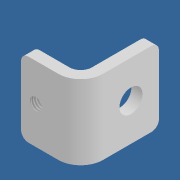
# Autodesk Inventor part: Belt_Tenshon
Saved by Autodesk Inventor 2020 (Build 240168000, 168)
## iProperties
Created: 2021-05-22
Part Number: Belt_Tenshon
Material: 一般
Document SubType Name: Sheet Metal
Designer: ken113
Density: 1 g/cm^3
Sheet Metal Rule: Default_mm
Appearance: 既定
Author: ken113
Autodesk Inventor part; units mm, degrees
ref_plane "YZ Plane" through (0, 0, 0) normal (1, 0, 0) x (0, 1, 0)
ref_plane "XZ Plane" through (0, 0, 0) normal (0, 1, 0) x (-1, 0, 0)
ref_plane "XY Plane" through (0, 0, 0) normal (0, 0, 1) x (1, 0, 0)
sketch "スケッチ1" plane through (0, 0, 0) normal (0, 0, 1) x (1, 0, 0)
  line L0 (-5, -10) -> (5, -10)
  line L1 (5, -10) -> (5, 10)
  line L2 (5, 10) -> (-5, 10)
  line L3 (-5, 10) -> (-5, -10)
  line L4 (-5, -10) -> (5, 10) construction
  line L5 (5, -10) -> (-5, 10) construction
  point P0 (0, 0)
  dimension "d0" = 10
  dimension "d1" = 20
  measures "d0" distance of L1.end L2.end
  measures "d1" distance of L2.end L0.start
extrude "プレート1" add sketch "スケッチ1" along normal blind 3
sketch "スケッチ2" plane through (8, -10, -3) normal (1, 0, 0) x (0, 1, 0)
  line L0 (20, 0) -> (0, 0)
  line L1 (0, 0) -> (0, -15)
  line L2 (0, -15) -> (20, -15)
  line L3 (20, -15) -> (20, 0)
  constraints: 6 end point, 1 horizontal, 1 perpendicular, 1 vertical
edge flange "フランジ1" height 21 angle 90 thickness 3 bend radius 3 thickness toward (1, 0, 0) relief straight relief width 3 relief depth 1.5 edges at (5, 0, 0) wall of the first edge with corners at (8, 10, -3) (8, -10, -3) (8, -10, -18) (8, 10, -18)
bend "曲げ1"
corner "コーナー1"
sketch "スケッチ3" plane through (0, 0, 3) normal (0, 0, 1) x (1, 0, 0)
  line L0 (-5, -10) -> (-5, 10) projected
  line L1 (5, -10) -> (-5, -10) projected
  line L2 (5, 10) -> (5, -10) projected
  line L3 (-5, 10) -> (5, 10) projected
  point P0 (-1, 0)
  dimension "d29" = 4
  measures "d29" distance from line of point (-1, 0) L0
hole "穴1" at (-1, 0, 3) direction (0, 0, -1) diameter 3.242 end through all thread size "M4x0.7" class "6H" standard "ISO Metric profile"
sketch "スケッチ4" plane through (11, -10, -18) normal (1, 0, 0) x (0, 0, -1)
  line L0 (-15, 20) -> (-15, 0) projected
  line L1 (0, 0) -> (-15, 0) projected
  line L2 (0, 20) -> (0, 0) projected
  line L3 (-15, 20) -> (0, 20) projected
  point P0 (-18, 10)
  point P1 (-7.5, 10)
  dimension "d20" = 7.5
  measures "d20" distance from line of L2 point (-7.5, 10)
hole "穴2" at (11, 0, -10.5) direction (-1, 0, 0) diameter 6.2 end through all
fillet "フィレット1" radius 2 4 edges at (-5, 10, 1.5) (-5, -10, 1.5) (9.5, 10, -18) (9.5, -10, -18)
equation "\"d2\" = Thickness"
equation "\"d3\" = BendReliefWidth"
equation "\"d4\" = BendReliefDepth"
equation "\"d5\" = MinimumRemnant"
equation "\"d6\" = TransitionRadius"
equation "\"d9\" = BendRadius"
equation "\"d10\" = CornerReliefSize"
equation "\"d11\" = GapSize"
equation "\"d12\" = JacobiRadiusSize"
equation "\"BendRadius\" = Thickness"
equation "\"BendReliefWidth\" = Thickness"
equation "\"BendReliefDepth\" = 0.5 * Thickness"
equation "\"CornerReliefSize\" = 4 * Thickness"
equation "\"MinimumRemnant\" = 2 * Thickness"
equation "\"TransitionRadius\" = BendRadius"
equation "\"JacobiRadiusSize\" = BendRadius"
equation "\"GapSize\" = Thickness"
equation "\"Thickness\" = 3"
